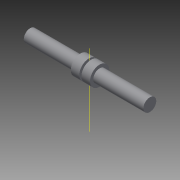
# Autodesk Inventor part: Top Axle
Saved by Autodesk Inventor 2015 (Build 190159000, 159)
## iProperties
Created: 2016-02-06
Part Number: Top Axle
Material: Generic
Document SubType Name: Modeling
Designer: sethbattis
Density: 1 g/cm^3
Appearance: Default
Author: sethbattis
Autodesk Inventor part; units mm, degrees
sketch "Sketch1" plane through (0, 0, 0) normal (1, 0, 0) x (0, 1, 0)
  circle A0 centre (0, 0) radius 9.525
  dimension "d0" = 19.05
  constraints: 1 centre point, 1 coincident
  measures "d0" diameter of A0
extrude "Extrusion1" add sketch "Sketch1" along normal blind 177.8
sketch "Sketch2" plane through (0, 0, 0) normal (0, 0, 1) x (1, 0, 0)
  line L0 (0, 9.525) -> (0, -9.525) projected
  line L1 (177.8, -9.525) -> (177.8, 9.525) projected
  line L2 (177.8, 0) -> (203.2, 0)
  line L3 (191.0369, -3.6537) -> (215.3631, 3.6537)
  line L4 (0, 0) -> (-25.4, 0)
  line L5 (-37.5631, 3.6537) -> (-13.2369, -3.6537)
  line L6 (-37.5631, 3.6537) -> (215.3631, 3.6537) construction
  line L7 (191.0369, -3.6537) -> (-13.2369, -3.6537) construction
  dimension "d3" = 25.4
  dimension "d4" = 16.72
  constraints: 12 end point, 3 equal length, 3 horizontal, 3 midpoint, 1 parallel
  measures "d3" distance of L2.end L2.start
  measures "d4" angle of L3 L2
ref_plane "Work Plane1" through (88.9, 0, 0) normal (1, 0, 0) x (0, 0, -1)
sketch "Sketch4" plane through (88.9, 0, 0) normal (1, 0, 0) x (0, 0, -1)
  circle A0 centre (0, 0) radius 14.2875
  dimension "d5" = 28.575
  constraints: 1 centre point, 1 coincident
  measures "d5" diameter of A0
extrude "Extrusion2" add sketch "Sketch4" along normal mid plane 28.575
sketch "Sketch5" plane through (88.9, 0, 0) normal (1, 0, 0) x (0, 0, -1)
  circle A0 centre (0, 0) radius 14.2875
  constraints: 1 centre point, 1 coincident
extrude "Extrusion3" cut sketch "Sketch5" along normal mid plane 3.175
sketch "Sketch6" plane through (0, 0, 0) normal (0, 1, 0) x (-1, 0, 0)
  line L0 (25.4, 0) -> (25.4, -14.6229)
  line L1 (-203.2, 0) -> (-203.2, -14.6229)
  point P0 (0, 0)
  constraints: 4 end point, 2 vertical
ref_plane "Work Plane2" through (203.2, 0, -14.6229) normal (-0.2877, 0.9577, 0) x (0, 0, 1)
sketch "Sketch7" plane through (203.2, 0, -14.6229) normal (-0.2877, 0.9577, 0) x (0, 0, 1)
  line L0 (9.6135, 0) -> (20.0925, 0)
  point P0 (14.6229, -194.6091)
  point P1 (14.6229, 0)
  constraints: 2 end point, 1 horizontal, 1 point on line
ref_plane "Work Plane4" through (-37.5631, 3.6537, 0) normal (0.2877, 0.9577, 0) x (0.9577, -0.2877, 0)
sketch "Sketch8" plane through (-37.5631, 3.6537, 0) normal (0.2877, 0.9577, 0) x (0.9577, -0.2877, 0)
  line L0 (12.7, 14.543) -> (12.7, -14.441)
  point P0 (37.0261, 0)
  point P1 (12.7, 0)
  constraints: 2 end point, 1 point on line, 1 vertical
sketch "Sketch9" plane through (88.9, 0, 0) normal (1, 0, 0) x (0, 0, -1)
  line L0 (0, 18.8045) -> (0, -31.5137)
  point P0 (0, 0)
  constraints: 2 end point, 1 vertical
body "Solid1"
